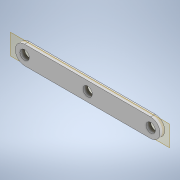
# Autodesk Inventor part: EslabonPreliminarElevacion
Saved by Autodesk Inventor 2021 (Build 250183000, 183)
## iProperties
Created: 2021-04-17
Part Number: EslabonPreliminarElevacion
Material: Generic
Document SubType Name: Modeling
Designer: GABRIEL LOL
Density: 1 g/cm^3
Appearance: Default
Mass: 111.142 g
Surface Area: 307.699 cm^2
Volume: 111.142 cm^3
Author: GABRIEL LOL
Autodesk Inventor part; units mm, degrees
ref_plane "YZ Plane" through (0, 0, 0) normal (1, 0, 0) x (0, 1, 0)
ref_plane "XZ Plane" through (0, 0, 0) normal (0, 1, 0) x (-1, 0, 0)
sketch "Sketch1" plane through (0, 0, 0) normal (0, 0, 1) x (1, 0, 0)
  line L0 (0, 0) -> (135, 0) construction
  line L1 (135, 0) -> (270, 0) construction
  circle A0 centre (0, 0) radius 10
  circle A1 centre (270, 0) radius 10
  circle A2 centre (0, 0) radius 20
  circle A3 centre (270, 0) radius 20
  line L2 (0, 20) -> (270, 20)
  line L3 (0, -20) -> (270, -20)
  circle A4 centre (135, 0) radius 10
  dimension "d0" = 135
  dimension "d1" = 20
  dimension "d2" = 20
  dimension "d3" = 40
  dimension "d4" = 40
  dimension "d7" = 20
  constraints: 8 end point, 5 centre point, 5 coincident, 4 point on circle, 2 horizontal, 2 tangent, 1 collinear, 1 point on line
  measures "d0" distance of L0.start L0.end
  measures "d1" diameter of A0
  measures "d2" diameter of A1
  measures "d3" diameter of A2
  measures "d4" diameter of A3
  measures "d7" diameter of A4
extrude "Extrusion1" add sketch "Sketch1" along normal blind 10
ref_plane "Work Plane1" through (0, 0, 5) normal (0, 0, 1) x (1, 0, 0)
body "Solid1"
